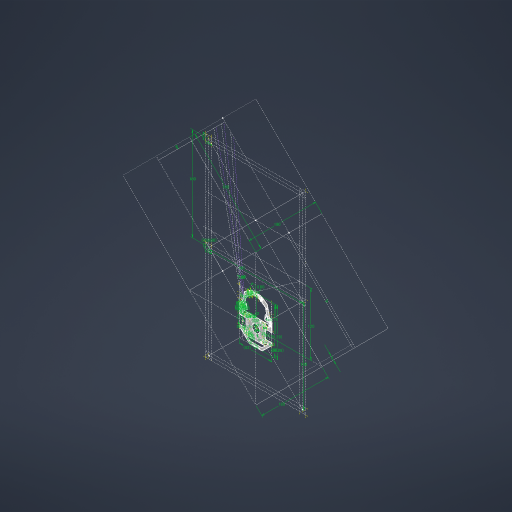
# Autodesk Inventor part: chassis
Saved by Autodesk Inventor 2023.5 (Build 275446000, 446)
## iProperties
Created: 2024-12-08
Part Number: chassis
Material: 一般
Document SubType Name: Modeling
Designer: IshiiLabHonda
Density: 1 g/cm^3
Appearance: 既定
Author: IshiiLabHonda
Autodesk Inventor part; units mm, degrees
(part 1 of 2)
ref_plane "YZ Plane" through (0, 0, 0) normal (1, 0, 0) x (0, 1, 0)
ref_plane "XZ Plane" through (0, 0, 0) normal (0, 1, 0) x (-1, 0, 0)
ref_plane "XY Plane" through (0, 0, 0) normal (0, 0, 1) x (1, 0, 0)
sketch "スケッチ1" plane through (0, 0, 0) normal (0, 0, 1) x (1, 0, 0)
  line L0 (0, 0) -> (0, 1) construction
  line L1 (0, 0) -> (1, 0) construction
  line L2 (-90, 90) -> (90, 90) construction
  line L3 (90, 90) -> (90, -90) construction
  line L4 (90, -90) -> (-90, -90) construction
  line L5 (-90, -90) -> (-90, 90) construction
  line L6 (-90, -90) -> (90, 90) construction
  line L7 (-90, 90) -> (90, -90) construction
  line L8 (-84, 96) -> (-84, 84) construction
  line L9 (-84, 84) -> (-96, 84) construction
  line L10 (-96, 84) -> (-96, 96) construction
  line L11 (-96, 96) -> (-84, 84) construction
  line L12 (-84, 96) -> (-96, 84) construction
  line L13 (-96, 96) -> (-84, 96) construction
  line L14 (-96, -96) -> (-96, -84) construction
  line L15 (-84, -96) -> (-96, -96) construction
  line L16 (-96, -96) -> (-84, -84) construction
  line L17 (-96, -84) -> (-84, -96) construction
  line L18 (-84, -84) -> (-84, -96) construction
  line L19 (-96, -84) -> (-84, -84) construction
  line L20 (96, -96) -> (84, -96) construction
  line L21 (96, -84) -> (96, -96) construction
  line L22 (96, -96) -> (84, -84) construction
  line L23 (84, -96) -> (96, -84) construction
  line L24 (84, -84) -> (96, -84) construction
  line L25 (84, -96) -> (84, -84) construction
  line L26 (96, 96) -> (96, 84) construction
  line L27 (84, 96) -> (96, 96) construction
  line L28 (96, 96) -> (84, 84) construction
  line L29 (96, 84) -> (84, 96) construction
  line L30 (84, 84) -> (84, 96) construction
  line L31 (96, 84) -> (84, 84) construction
  line L32 (-84, 84) -> (-84, -84) construction
  line L33 (-96, 84) -> (-96, -84) construction
  line L34 (-84, -84) -> (84, -84) construction
  line L35 (-84, -96) -> (84, -96) construction
  line L36 (96, 84) -> (96, -84) construction
  line L37 (84, 84) -> (84, -84) construction
  line L38 (-84, 96) -> (84, 96) construction
  line L39 (-84, 84) -> (84, 84) construction
  line L40 (-19, 15) -> (19, 15) construction
  line L41 (19, 15) -> (19, -15) construction
  line L42 (19, -15) -> (-19, -15) construction
  line L43 (-19, -15) -> (-19, 15) construction
  line L44 (-19, 15) -> (19, -15) construction
  line L45 (19, 15) -> (-19, -15) construction
  line L46 (-30.25, 11.5) -> (-19, 11.5) construction
  line L47 (-19, -11.5) -> (-30.25, -11.5) construction
  line L48 (-30.25, -11.5) -> (-30.25, 11.5) construction
  line L49 (-30.25, 11.5) -> (-19, -11.5) construction
  line L50 (-19, 11.5) -> (-30.25, -11.5) construction
  line L51 (30.25, 11.5) -> (19, 11.5) construction
  line L52 (19, -11.5) -> (30.25, -11.5) construction
  line L53 (30.25, -11.5) -> (30.25, 11.5) construction
  line L54 (30.25, 11.5) -> (19, -11.5) construction
  line L55 (19, 11.5) -> (30.25, -11.5) construction
  line L56 (-19, -10) -> (19, -10) construction
  line L57 (-19, -12.5) -> (19, -12.5) construction
  line L58 (-19, 10) -> (19, 10) construction
  line L59 (-19, 12.5) -> (19, 12.5) construction
  line L60 (-16.5, -15) -> (-16.5, 15) construction
  line L61 (16.5, -15) -> (16.5, 15) construction
  line L62 (-12.5, -10) -> (-12.5, -15) construction
  line L63 (-16.5, -10) -> (-12.5, -15) construction
  line L64 (-16.5, -15) -> (-12.5, -10) construction
  circle A0 centre (-14.5, -12.5) radius 0.8 construction
  line L65 (12.5, -10) -> (12.5, -15) construction
  line L66 (16.5, -10) -> (12.5, -15) construction
  line L67 (16.5, -15) -> (12.5, -10) construction
  circle A1 centre (14.5, -12.5) radius 0.8 construction
  line L68 (-12.5, 10) -> (-12.5, 15) construction
  line L69 (-16.5, 10) -> (-12.5, 15) construction
  line L70 (-16.5, 15) -> (-12.5, 10) construction
  circle A2 centre (-14.5, 12.5) radius 0.8 construction
  line L71 (12.5, 10) -> (12.5, 15) construction
  line L72 (16.5, 10) -> (12.5, 15) construction
  circle A3 centre (14.5, 12.5) radius 0.8 construction
  line L73 (16.5, 15) -> (12.5, 10) construction
  line L74 (-96, 276) -> (-84, 276) construction
  line L75 (-84, 276) -> (-84, 264) construction
  line L76 (-84, 264) -> (-96, 264) construction
  line L77 (-96, 264) -> (-96, 276) construction
  line L78 (-96, 276) -> (-84, 264) construction
  line L79 (-84, 276) -> (-96, 264) construction
  line L80 (-90, 90) -> (-90, 270) construction
  line L81 (-96, 264) -> (-96, 96) construction
  line L82 (-84, 264) -> (-84, 96) construction
  line L83 (96, 276) -> (84, 276) construction
  line L84 (84, 276) -> (84, 264) construction
  line L85 (84, 264) -> (96, 264) construction
  line L86 (96, 264) -> (96, 276) construction
  line L87 (96, 276) -> (84, 264) construction
  line L88 (84, 276) -> (96, 264) construction
  line L89 (90, 90) -> (90, 270) construction
  line L90 (96, 264) -> (96, 96) construction
  line L91 (84, 264) -> (84, 96) construction
  line L92 (-84, 276) -> (84, 276) construction
  line L93 (-84, 264) -> (84, 264) construction
  line L94 (-90, 270) -> (90, 270) construction
  line L95 (-90, 270) -> (90, 90) construction
  line L96 (-90, 90) -> (90, 270) construction
  circle A4 centre (0, 0) radius 15 construction
  line L97 (-96, 120) -> (96, 120) construction
  line L98 (0, 127.2792) -> (0, -127.2792) construction
  line L99 (-127.2792, 0) -> (127.2792, 0) construction
  line L100 (127.2792, 0) -> (0, -127.2792) construction
  line L101 (0, -127.2792) -> (-127.2792, 0) construction
  line L102 (-127.2792, 0) -> (0, 127.2792) construction
  line L103 (0, 127.2792) -> (127.2792, 0) construction
  line L104 (127.2792, 254.5584) -> (254.5584, 127.2792) construction
  line L105 (254.5584, 127.2792) -> (127.2792, 0) construction
  line L106 (127.2792, 0) -> (0, 127.2792) construction
  line L107 (0, 127.2792) -> (127.2792, 254.5584) construction
  line L108 (-127.2792, 254.5584) -> (0, 127.2792) construction
  line L109 (0, 127.2792) -> (-127.2792, 0) construction
  line L110 (-127.2792, 0) -> (-254.5584, 127.2792) construction
  line L111 (-254.5584, 127.2792) -> (-127.2792, 254.5584) construction
  line L112 (0, 381.8377) -> (127.2792, 254.5584) construction
  line L113 (127.2792, 254.5584) -> (0, 127.2792) construction
  line L114 (0, 127.2792) -> (-127.2792, 254.5584) construction
  line L115 (-127.2792, 254.5584) -> (0, 381.8377) construction
  line L116 (190.9188, 63.6396) -> (63.6396, 190.9188) construction
  line L117 (-190.9188, 190.9188) -> (-63.6396, 63.6396) construction
  line L118 (59.397, -59.397) -> (186.6762, 67.8823) construction
  line L119 (59.397, 186.6762) -> (186.6762, 59.397) construction
  line L120 (63.6396, 190.9188) -> (-63.6396, 318.1981) construction
  line L121 (-186.6762, 186.6762) -> (-59.397, 313.9554) construction
  point P0 (-90, -90)
  point P1 (90, -90)
  point P2 (-24.625, 0)
  point P3 (-84, 120)
  point P4 (84, 120)
  point P5 (0, 0)
  dimension "d0" = 1
  dimension "d1" = 1
  dimension "d2" = 180
  dimension "d3" = 180
  dimension "d4" = 12
  dimension "d5" = 12
  dimension "d8" = 360
  dimension "d10" = 38
  dimension "d12" = 11.25
  dimension "d13" = 23
  dimension "d14" = 5
  dimension "d15" = 2.5
  dimension "d16" = 4
  dimension "d17" = 1.6
  dimension "d22" = 12
  dimension "d23" = 12
  dimension "d24" = 180
  dimension "d25" = 25
  dimension "d26" = 30
  dimension "d27" = 30
  dimension "d29" = 120
  dimension "d331" = 180
  dimension "d334" = 180
  dimension "d337" = 180
  dimension "d340" = 6
  dimension "d341" = 6
  dimension "d342" = 6
  constraints: 244 end point, 29 point on line, 27 symmetric about line, 19 midpoint, 18 parallel, 10 perpendicular, 5 centre point, 4 coincident, 2 collinear, 1 horizontal, 1 vertical, 91 other
  measures "d0" distance of L0.start L0.end
  measures "d1" distance of L0.start L1.end
  measures "d2" distance of L2.start L2.end
  measures "d3" distance of L2.end L3.end
  measures "d4" distance of L9.end L10.end
  measures "d5" distance of L8.end L9.end
  measures "d10" distance of L40.start L40.end
  measures "d12" distance of L46.start L46.end
  measures "d13" distance of L47.end L46.start
  measures "d14" distance between parallel lines of L56 L42
  measures "d15" distance between parallel lines of L43 L60
  measures "d16" distance between parallel lines of L60 L62
  measures "d17" diameter of A0
  measures "d22" distance of L75.end L76.end
  measures "d23" distance of L76.end L74.start
  measures "d24" distance of L2.start L80.end
  measures "d25" distance between parallel lines of L57 L59
  measures "d26" distance between parallel lines of L42 L40
  measures "d27" diameter of A4
  measures "d29" distance between parallel lines of L1 L97
  measures "d331" distance of L100.start L100.end
  measures "d334" distance of L102.end L104.start
  measures "d337" distance of L102.end L108.start
  measures "d340" distance between parallel lines of L118 L105
  measures "d341" distance between parallel lines of L116 L119
  measures "d342" distance between parallel lines of L111 L121
sketch "スケッチ4" plane through (0, 0, 0) normal (0, 0, 1) x (1, 0, 0)
  line L0 (-84, 264) -> (-96, 264) construction
  line L1 (-90, 90) -> (-90, 270) construction
  line L2 (-96, 264) -> (-96, 96) construction
  line L3 (-96, 96) -> (-84, 96) construction
  line L4 (-84, 96) -> (-84, 84) construction
  line L5 (-84, 96) -> (-96, 84) construction
  line L6 (-96, 96) -> (-84, 84) construction
  line L7 (-84, 264) -> (-84, 96) construction
  line L8 (-84, 84) -> (-96, 84) construction
  line L9 (84, -84) -> (96, -84) construction
  line L10 (84, -96) -> (96, -84) construction
  line L11 (96, -96) -> (84, -84) construction
  line L12 (96, -84) -> (96, -96) construction
  line L13 (96, -96) -> (84, -96) construction
  line L14 (0, 0) -> (0, 1) construction
  line L15 (0, 0) -> (1, 0) construction
  line L16 (16.5, 15) -> (12.5, 10) construction
  line L17 (-96, 84) -> (-96, -84) construction
  line L18 (-84, 84) -> (-84, -84) construction
  line L19 (-90, -90) -> (-90, 90) construction
  line L20 (-90, 90) -> (90, 90) construction
  line L21 (-84, -84) -> (84, -84) construction
  line L22 (-84, -96) -> (84, -96) construction
  line L23 (-90, -90) -> (90, 90) construction
  line L24 (90, -90) -> (-90, -90) construction
  line L25 (-90, 90) -> (90, -90) construction
  line L26 (84, 84) -> (84, -84) construction
  line L27 (90, 90) -> (90, -90) construction
  line L28 (96, 84) -> (96, -84) construction
  line L29 (-96, 84) -> (-96, 96) construction
  line L30 (-84, -84) -> (-84, -96) construction
  line L31 (-96, -84) -> (-84, -84) construction
  line L32 (-84, -96) -> (-96, -96) construction
  line L33 (-96, -96) -> (-84, -84) construction
  line L34 (-96, -84) -> (-84, -96) construction
  line L35 (-96, -96) -> (-96, -84) construction
  line L36 (84, -96) -> (84, -84) construction
  line L37 (-19, -15) -> (-19, 15) construction
  line L38 (-30.25, 11.5) -> (-19, 11.5) construction
  line L39 (-19, -11.5) -> (-30.25, -11.5) construction
  line L40 (-19, 11.5) -> (-30.25, -11.5) construction
  line L41 (-30.25, 11.5) -> (-19, -11.5) construction
  line L42 (-30.25, -11.5) -> (-30.25, 11.5) construction
  line L43 (12.5, 10) -> (12.5, 15) construction
  circle A0 centre (14.5, 12.5) radius 0.8 construction
  line L44 (30.25, 11.5) -> (19, 11.5) construction
  line L45 (16.5, 10) -> (12.5, 15) construction
  circle A1 centre (14.5, -12.5) radius 0.8 construction
  line L46 (16.5, -15) -> (12.5, -10) construction
  line L47 (16.5, -10) -> (12.5, -15) construction
  line L48 (12.5, -10) -> (12.5, -15) construction
  circle A2 centre (-14.5, -12.5) radius 0.8 construction
  line L49 (-12.5, -10) -> (-12.5, -15) construction
  line L50 (-16.5, -15) -> (-12.5, -10) construction
  line L51 (-16.5, -10) -> (-12.5, -15) construction
  line L52 (96, 84) -> (84, 84) construction
  line L53 (96, 96) -> (96, 84) construction
  line L54 (84, 96) -> (96, 96) construction
  line L55 (96, 96) -> (84, 84) construction
  line L56 (84, 84) -> (84, 96) construction
  line L57 (96, 84) -> (84, 96) construction
  line L58 (-96, 264) -> (-96, 276) construction
  line L59 (-84, 276) -> (-84, 264) construction
  line L60 (-96, 276) -> (-84, 276) construction
  line L61 (-96, 276) -> (-84, 264) construction
  line L62 (-84, 276) -> (-96, 264) construction
  line L63 (-84, 84) -> (84, 84) construction
  line L64 (-84, 96) -> (84, 96) construction
  line L65 (84, 264) -> (84, 96) construction
  line L66 (90, 90) -> (90, 270) construction
  line L67 (-90, 90) -> (90, 270) construction
  line L68 (-90, 270) -> (90, 90) construction
  line L69 (96, 264) -> (96, 96) construction
  line L70 (-96, 120) -> (96, 120) construction
  line L71 (-84, 264) -> (84, 264) construction
  line L72 (-84, 276) -> (84, 276) construction
  line L73 (-90, 270) -> (90, 270) construction
  line L74 (84, 276) -> (84, 264) construction
  line L75 (84, 264) -> (96, 264) construction
  line L76 (96, 264) -> (96, 276) construction
  line L77 (96, 276) -> (84, 264) construction
  line L78 (96, 276) -> (84, 276) construction
  line L79 (84, 276) -> (96, 264) construction
  line L80 (-19, 15) -> (19, 15) construction
  line L81 (19, 15) -> (19, -15) construction
  line L82 (19, -15) -> (-19, -15) construction
  circle A3 centre (-14.5, 12.5) radius 0.8 construction
  line L83 (-16.5, 10) -> (-12.5, 15) construction
  line L84 (-12.5, 10) -> (-12.5, 15) construction
  line L85 (-16.5, 15) -> (-12.5, 10) construction
  circle A4 centre (0, 0) radius 15 construction
  line L86 (-19, 10) -> (19, 10) construction
  line L87 (-19, 12.5) -> (19, 12.5) construction
  line L88 (-19, 15) -> (19, -15) construction
  line L89 (19, 15) -> (-19, -15) construction
  line L90 (-19, -10) -> (19, -10) construction
  line L91 (-19, -12.5) -> (19, -12.5) construction
  line L92 (16.5, -15) -> (16.5, 15) construction
  line L93 (19, 11.5) -> (30.25, -11.5) construction
  line L94 (19, -11.5) -> (30.25, -11.5) construction
  line L95 (30.25, -11.5) -> (30.25, 11.5) construction
  line L96 (30.25, 11.5) -> (19, -11.5) construction
  line L97 (-16.5, -15) -> (-16.5, 15) construction
  line L98 (-84, 120) -> (30.25, 40.0013) construction
  line L99 (84, 120) -> (-30.25, 40.0013) construction
  line L100 (-30.25, 57) -> (30.25, 57) construction
  line L101 (1.0005, 57) -> (-30.25, 35.1182) construction
  line L102 (-1.0005, 57) -> (30.25, 35.1182) construction
  line L103 (-12.9471, 57) -> (-30.25, 44.8844) construction
  line L104 (-10.2335, 58.2897) -> (-6.2185, 52.5556) construction
  line L105 (-6.2185, 52.5556) -> (-11.543, 48.8274) construction
  line L106 (-11.543, 48.8274) -> (-15.558, 54.5615) construction
  line L107 (-15.558, 54.5615) -> (-10.2335, 58.2897) construction
  line L108 (-10.2335, 58.2897) -> (-11.543, 48.8274) construction
  line L109 (-6.2185, 52.5556) -> (-15.558, 54.5615) construction
  line L110 (-9.6599, 57.4705) -> (-14.9844, 53.7423) construction
  line L111 (-6.7921, 53.3748) -> (-12.1165, 49.6465) construction
  line L112 (-10.8882, 53.5585) -> (-10.2329, 54.0174) construction
  line L113 (-10.8882, 53.5585) -> (-10.4294, 52.9032) construction
  line L114 (-10.5199, 55.6476) -> (-8.7991, 53.1902) construction
  line L115 (-8.7991, 53.1902) -> (-11.2566, 51.4694) construction
  line L116 (-11.2566, 51.4694) -> (-12.9773, 53.9269) construction
  line L117 (-12.9773, 53.9269) -> (-10.5199, 55.6476) construction
  line L118 (-10.5199, 55.6476) -> (-11.2566, 51.4694) construction
  line L119 (-8.7991, 53.1902) -> (-12.9773, 53.9269) construction
  circle A5 centre (-10.8882, 53.5585) radius 0.8 construction
  line L120 (-30.25, 11.5) -> (-30.25, 57) construction
  line L121 (30.25, 11.5) -> (30.25, 57) construction
  line L122 (-6.1403, 52) -> (6.1403, 52) construction
  line L123 (-31, 57) -> (-31, -31) construction
  line L124 (31, 57) -> (31, -31) construction
  line L125 (-30.25, 57) -> (-31, 57) construction
  line L126 (30.25, 57) -> (31, 57) construction
  line L127 (-31, 8.5) -> (31, 8.5) construction
  line L128 (-31, -8.5) -> (31, -8.5) construction
  circle A6 centre (0, 0) radius 7.5 construction
  line L129 (-31, -31) -> (31, -31) construction
  line L130 (-30.25, 44.8844) -> (-31, 44.3592) construction
  line L131 (-30.25, 35.1182) -> (-31, 34.593) construction
  line L132 (-26.25, 26.5) -> (-26.3613, 27.2922) construction
  line L133 (-26.25, 26.5) -> (-25.4578, 26.6113) construction
  line L134 (-29.0736, 28.6277) -> (-24.1223, 29.3236) construction
  line L135 (-24.1223, 29.3236) -> (-23.4264, 24.3723) construction
  line L136 (-23.4264, 24.3723) -> (-28.3777, 23.6764) construction
  line L137 (-28.3777, 23.6764) -> (-29.0736, 28.6277) construction
  line L138 (-29.0736, 28.6277) -> (-23.4264, 24.3723) construction
  line L139 (-24.1223, 29.3236) -> (-28.3777, 23.6764) construction
  circle A7 centre (-26.25, 26.5) radius 0.8 construction
  line L140 (-26.25, 57) -> (-26.25, -31) construction
  line L141 (-96, 180) -> (96, 180) construction
  line L142 (-26.3613, 27.2922) -> (-65.7556, 307.5968) construction
  line L143 (-186.6762, 186.6762) -> (-59.397, 313.9554) construction
  line L144 (59.397, 186.6762) -> (186.6762, 59.397) construction
  line L145 (-26.25, 26.5) -> (-80.4501, 292.9022) construction
  line L146 (-26.25, 26.5) -> (-47.9742, 302.5327) construction
  line L147 (63.6396, 190.9188) -> (-63.6396, 318.1981) construction
  line L148 (10.2335, 58.2897) -> (6.2185, 52.5556) construction
  line L149 (6.2185, 52.5556) -> (11.543, 48.8274) construction
  line L150 (11.543, 48.8274) -> (15.558, 54.5615) construction
  line L151 (15.558, 54.5615) -> (10.2335, 58.2897) construction
  line L152 (10.2335, 58.2897) -> (11.543, 48.8274) construction
  line L153 (6.2185, 52.5556) -> (15.558, 54.5615) construction
  line L154 (9.6599, 57.4705) -> (14.9844, 53.7423) construction
  line L155 (6.7921, 53.3748) -> (12.1165, 49.6465) construction
  line L156 (10.8882, 53.5585) -> (10.2329, 54.0174) construction
  line L157 (10.8882, 53.5585) -> (10.4294, 52.9032) construction
  line L158 (10.5199, 55.6476) -> (8.7991, 53.1902) construction
  line L159 (8.7991, 53.1902) -> (11.2566, 51.4694) construction
  line L160 (11.2566, 51.4694) -> (12.9773, 53.9269) construction
  line L161 (12.9773, 53.9269) -> (10.5199, 55.6476) construction
  line L162 (10.5199, 55.6476) -> (11.2566, 51.4694) construction
  line L163 (8.7991, 53.1902) -> (12.9773, 53.9269) construction
  circle A8 centre (10.8882, 53.5585) radius 0.8 construction
  line L164 (-24.1223, 29.3236) -> (-19.1709, 30.0195) construction
  line L165 (-19.1709, 30.0195) -> (-18.4751, 25.0681) construction
  line L166 (-18.4751, 25.0681) -> (-23.4264, 24.3723) construction
  line L167 (-24.1223, 29.3236) -> (-29.0736, 28.6277) construction
  line L168 (-29.0736, 28.6277) -> (-28.3777, 23.6764) construction
  line L169 (-28.3777, 23.6764) -> (-23.4264, 24.3723) construction
  line L170 (28.3777, 23.6764) -> (29.0736, 28.6277) construction
  line L171 (24.1223, 29.3236) -> (19.1709, 30.0195) construction
  line L172 (19.1709, 30.0195) -> (18.4751, 25.0681) construction
  line L173 (18.4751, 25.0681) -> (23.4264, 24.3723) construction
  line L174 (24.1223, 29.3236) -> (29.0736, 28.6277) construction
  line L175 (29.0736, 28.6277) -> (28.3777, 23.6764) construction
  line L176 (28.3777, 23.6764) -> (23.4264, 24.3723) construction
  line L177 (24.1223, 29.3236) -> (28.3777, 23.6764) construction
  line L178 (23.4264, 24.3723) -> (29.0736, 28.6277) construction
  line L179 (-21.2987, 27.1959) -> (-61.3286, 312.0238) construction
  line L180 (-21.2987, 27.1959) -> (-76.2182, 297.1342) construction
  line L181 (-21.2987, 27.1959) -> (-42.5405, 297.0989) construction
  line L182 (-24.1223, 29.3236) -> (-18.4751, 25.0681) construction
  line L183 (-23.4264, 24.3723) -> (-19.1709, 30.0195) construction
  line L184 (-15.558, 54.5615) -> (-18.0155, 52.8407) construction
  line L185 (-18.0155, 52.8407) -> (-14.0004, 47.1067) construction
  line L186 (-14.0004, 47.1067) -> (-11.543, 48.8274) construction
  point P0 (90, -90)
  point P1 (-90, -90)
  point P2 (-24.625, 0)
  point P3 (0, 61.1826)
  point P4 (-5.9733, 57)
  point P5 (-8.226, 55.4227)
  point P6 (0, 180)
  point P7 (8.226, 55.4227)
  dimension "d264" = 110
  dimension "d275" = 7
  dimension "d276" = 6.5
  dimension "d277" = 5
  dimension "d278" = 3
  dimension "d279" = 3
  dimension "d280" = 1.6
  dimension "d281" = 8
  dimension "d284" = 5
  dimension "d288" = 17
  dimension "d289" = 15
  dimension "d290" = 0.75
  dimension "d291" = 0.75
  dimension "d292" = 88
  dimension "d296" = 5
  dimension "d297" = 5
  dimension "d298" = 1.6
  dimension "d299" = 8
  dimension "d345" = 7
  dimension "d346" = 15
  dimension "d356" = 16
  dimension "d367" = 4
  dimension "d369" = 42
  dimension "d370" = 6
  dimension "d371" = 62
  dimension "d382" = 5
  dimension "d385" = 7
  dimension "d513" = 3
  constraints: 172 end point, 38 point on line, 25 symmetric about line, 19 parallel, 15 perpendicular, 13 midpoint, 6 point on circle, 5 collinear, 4 centre point, 4 coincident, 2 equal length, 8 other
  measures "d264" angle of L99 L98
  measures "d275" distance of L104.start L104.end
  measures "d276" distance of L106.end L104.start
  measures "d277" distance between parallel lines of L110 L111
  measures "d278" distance of L115.end L116.end
  measures "d279" distance of L114.end L115.end
  measures "d280" diameter of A5
  measures "d281" distance between parallel lines of L101 L103
  measures "d284" distance between parallel lines of L100 L122
  measures "d288" distance between parallel lines of L128 L127
  measures "d289" diameter of A6
  measures "d290" distance between parallel lines of L123 L120
  measures "d291" distance between parallel lines of L121 L124
  measures "d292" distance between parallel lines of L129 L100
  measures "d296" distance of L135.end L136.end
  measures "d297" distance of L134.end L135.end
  measures "d298" diameter of A7
  measures "d299" angle of L140 L132
  measures "d345" angle of L145 L146
  measures "d346" distance from line of L38 L132.start
  measures "d356" distance between parallel lines of L129 L82
  measures "d367" distance between parallel lines of L120 L140
  measures "d369" distance between parallel lines of L80 L100
  measures "d370" distance of L112.start point (-5.973, 57)
  measures "d371" distance of L123.end L124.end
  measures "d382" distance of L134.end L164.end
  measures "d385" angle of L180 L181
  measures "d513" distance between parallel lines of L185 L106
sketch "スケッチ5" plane through (0, 0, 0) normal (0, 0, 1) x (1, 0, 0)
  line L0 (0, 0) -> (0, 1) construction
  line L1 (30.25, 11.5) -> (19, 11.5) construction
  line L2 (19, 11.5) -> (30.25, -11.5) construction
  line L3 (30.25, 11.5) -> (19, -11.5) construction
  line L4 (30.25, -11.5) -> (30.25, 11.5) construction
  line L5 (19, -11.5) -> (30.25, -11.5) construction
  line L6 (-90, 90) -> (90, 90) construction
  line L7 (-90, -90) -> (90, 90) construction
  line L8 (-90, 90) -> (90, -90) construction
  line L9 (-84, 84) -> (-84, -84) construction
  line L10 (-96, 84) -> (-96, -84) construction
  line L11 (-90, -90) -> (-90, 90) construction
  line L12 (-84, 84) -> (-96, 84) construction
  line L13 (-96, 84) -> (-96, 96) construction
  line L14 (84, 84) -> (84, -84) construction
  line L15 (90, 90) -> (90, -90) construction
  line L16 (96, 84) -> (84, 84) construction
  line L17 (96, 84) -> (96, -84) construction
  line L18 (90, -90) -> (-90, -90) construction
  line L19 (-84, -84) -> (84, -84) construction
  line L20 (-84, -96) -> (84, -96) construction
  line L21 (-84, -84) -> (-84, -96) construction
  line L22 (-96, -96) -> (-96, -84) construction
  line L23 (-84, -96) -> (-96, -96) construction
  line L24 (-96, -96) -> (-84, -84) construction
  line L25 (-96, -84) -> (-84, -96) construction
  line L26 (-96, -84) -> (-84, -84) construction
  line L27 (0, 0) -> (1, 0) construction
  line L28 (-84, 264) -> (-96, 264) construction
  line L29 (-96, 276) -> (-84, 276) construction
  line L30 (-96, 264) -> (-96, 276) construction
  line L31 (-84, 276) -> (-96, 264) construction
  line L32 (-96, 276) -> (-84, 264) construction
  line L33 (-84, 276) -> (-84, 264) construction
  line L34 (84, -96) -> (84, -84) construction
  line L35 (96, -96) -> (84, -96) construction
  line L36 (96, -84) -> (96, -96) construction
  line L37 (96, -96) -> (84, -84) construction
  line L38 (84, -96) -> (96, -84) construction
  line L39 (84, -84) -> (96, -84) construction
  line L40 (-19, 15) -> (19, 15) construction
  line L41 (19, 15) -> (19, -15) construction
  line L42 (16.5, 15) -> (12.5, 10) construction
  line L43 (12.5, 10) -> (12.5, 15) construction
  line L44 (16.5, 10) -> (12.5, 15) construction
  line L45 (16.5, -15) -> (16.5, 15) construction
  line L46 (-19, 10) -> (19, 10) construction
  line L47 (-19, 12.5) -> (19, 12.5) construction
  circle A0 centre (0, 0) radius 15 construction
  line L48 (-19, -10) -> (19, -10) construction
  line L49 (-19, -12.5) -> (19, -12.5) construction
  line L50 (19, -15) -> (-19, -15) construction
  line L51 (-19, 15) -> (19, -15) construction
  line L52 (19, 15) -> (-19, -15) construction
  line L53 (-16.5, -15) -> (-16.5, 15) construction
  line L54 (-19, -15) -> (-19, 15) construction
  line L55 (-30.25, 11.5) -> (-19, 11.5) construction
  line L56 (-19, -11.5) -> (-30.25, -11.5) construction
  line L57 (-30.25, -11.5) -> (-30.25, 11.5) construction
  line L58 (-30.25, 11.5) -> (-19, -11.5) construction
  line L59 (-19, 11.5) -> (-30.25, -11.5) construction
  line L60 (-12.5, 10) -> (-12.5, 15) construction
  circle A1 centre (-14.5, 12.5) radius 0.8 construction
  line L61 (-16.5, 10) -> (-12.5, 15) construction
  line L62 (-16.5, 15) -> (-12.5, 10) construction
  circle A2 centre (14.5, 12.5) radius 0.8 construction
  line L63 (-84, 96) -> (-96, 84) construction
  line L64 (-96, 96) -> (-84, 96) construction
  line L65 (-84, 96) -> (-84, 84) construction
  line L66 (-96, 96) -> (-84, 84) construction
  line L67 (-96, 264) -> (-96, 96) construction
  line L68 (-84, 264) -> (-84, 96) construction
  line L69 (-84, 96) -> (84, 96) construction
  line L70 (-84, 84) -> (84, 84) construction
  line L71 (84, 84) -> (84, 96) construction
  line L72 (96, 96) -> (96, 84) construction
  line L73 (96, 96) -> (84, 84) construction
  line L74 (96, 84) -> (84, 96) construction
  line L75 (-96, 120) -> (96, 120) construction
  line L76 (84, 96) -> (96, 96) construction
  line L77 (-84, 264) -> (84, 264) construction
  line L78 (84, 264) -> (84, 96) construction
  line L79 (-84, 276) -> (84, 276) construction
  line L80 (96, 264) -> (96, 96) construction
  line L81 (-90, 270) -> (90, 270) construction
  line L82 (-90, 270) -> (90, 90) construction
  line L83 (-90, 90) -> (90, 270) construction
  line L84 (90, 90) -> (90, 270) construction
  line L85 (-90, 90) -> (-90, 270) construction
  line L86 (84, 264) -> (96, 264) construction
  line L87 (96, 276) -> (84, 276) construction
  line L88 (96, 276) -> (84, 264) construction
  line L89 (84, 276) -> (96, 264) construction
  line L90 (96, 264) -> (96, 276) construction
  line L91 (84, 276) -> (84, 264) construction
  circle A3 centre (-14.5, -12.5) radius 0.8 construction
  line L92 (-12.5, -10) -> (-12.5, -15) construction
  line L93 (-16.5, -15) -> (-12.5, -10) construction
  line L94 (12.5, -10) -> (12.5, -15) construction
  circle A4 centre (14.5, -12.5) radius 0.8 construction
  line L95 (16.5, -15) -> (12.5, -10) construction
  line L96 (16.5, -10) -> (12.5, -15) construction
  line L97 (-16.5, -10) -> (-12.5, -15) construction
  line L98 (-12.9773, 53.9269) -> (-10.5199, 55.6476) construction
  line L99 (-8.7991, 53.1902) -> (-12.9773, 53.9269) construction
  circle A5 centre (-10.8882, 53.5585) radius 0.8 construction
  line L100 (-8.7991, 53.1902) -> (-11.2566, 51.4694) construction
  line L101 (-10.5199, 55.6476) -> (-11.2566, 51.4694) construction
  line L102 (-11.2566, 51.4694) -> (-12.9773, 53.9269) construction
  line L103 (-30.25, 44.8844) -> (-31, 44.3592) construction
  line L104 (-12.9471, 57) -> (-30.25, 44.8844) construction
  line L105 (-30.25, 57) -> (-31, 57) construction
  line L106 (-10.5199, 55.6476) -> (-8.7991, 53.1902) construction
  line L107 (-30.25, 57) -> (30.25, 57) construction
  line L108 (-6.2185, 52.5556) -> (-11.543, 48.8274) construction
  line L109 (-11.543, 48.8274) -> (-15.558, 54.5615) construction
  line L110 (-10.2335, 58.2897) -> (-6.2185, 52.5556) construction
  line L111 (1.0005, 57) -> (-30.25, 35.1182) construction
  line L112 (-1.0005, 57) -> (30.25, 35.1182) construction
  line L113 (-19, 15) -> (19, 15) construction
  line L114 (12.5, 10) -> (12.5, 15) construction
  line L115 (-19, 10) -> (19, 10) construction
  circle A6 centre (-14.5, 12.5) radius 0.8 construction
  line L116 (-12.5, 10) -> (-12.5, 15) construction
  line L117 (-16.5, 10) -> (-12.5, 15) construction
  line L118 (-16.5, 15) -> (-12.5, 10) construction
  line L119 (-19, 12.5) -> (19, 12.5) construction
  line L120 (30.25, 57) -> (31, 57) construction
  line L121 (30.25, 11.5) -> (30.25, 57) construction
  line L122 (-6.1403, 52) -> (6.1403, 52) construction
  line L123 (-30.25, 35.1182) -> (-31, 34.593) construction
  line L124 (-30.25, 11.5) -> (-30.25, 57) construction
  line L125 (-6.7921, 53.3748) -> (-12.1165, 49.6465) construction
  line L126 (-10.8882, 53.5585) -> (-10.4294, 52.9032) construction
  line L127 (-10.8882, 53.5585) -> (-10.2329, 54.0174) construction
  line L128 (-6.2185, 52.5556) -> (-15.558, 54.5615) construction
  line L129 (-9.6599, 57.4705) -> (-14.9844, 53.7423) construction
  line L130 (-15.558, 54.5615) -> (-10.2335, 58.2897) construction
  line L131 (-10.2335, 58.2897) -> (-11.543, 48.8274) construction
  line L132 (-30.25, 11.5) -> (-19, 11.5) construction
  line L133 (-30.25, 11.5) -> (-19, -11.5) construction
  line L134 (30.25, 11.5) -> (19, 11.5) construction
  line L135 (30.25, -11.5) -> (30.25, 11.5) construction
  line L136 (19, 11.5) -> (30.25, -11.5) construction
  line L137 (30.25, 11.5) -> (19, -11.5) construction
  line L138 (0, 0) -> (0, 1) construction
  line L139 (0, 0) -> (1, 0) construction
  circle A7 centre (0, 0) radius 7.5 construction
  circle A8 centre (0, 0) radius 15 construction
  line L140 (-16.5, -15) -> (-16.5, 15) construction
  circle A9 centre (14.5, 12.5) radius 0.8 construction
  line L141 (-12.5, -10) -> (-12.5, -15) construction
  line L142 (12.5, -10) -> (12.5, -15) construction
  line L143 (16.5, 10) -> (12.5, 15) construction
  line L144 (-16.5, -15) -> (-12.5, -10) construction
  line L145 (16.5, -10) -> (12.5, -15) construction
  line L146 (16.5, 15) -> (12.5, 10) construction
  line L147 (-19, -12.5) -> (19, -12.5) construction
  line L148 (19, -15) -> (-19, -15) construction
  line L149 (-19, 11.5) -> (-30.25, -11.5) construction
  line L150 (19, -11.5) -> (30.25, -11.5) construction
  line L151 (-19, -11.5) -> (-30.25, -11.5) construction
  line L152 (-30.25, -11.5) -> (-30.25, 11.5) construction
  line L153 (16.5, -15) -> (16.5, 15) construction
  line L154 (19, 15) -> (19, -15) construction
  line L155 (-19, -15) -> (-19, 15) construction
  line L156 (-19, 15) -> (19, -15) construction
  line L157 (19, 15) -> (-19, -15) construction
  line L158 (-31, -8.5) -> (31, -8.5) construction
  line L159 (-31, 8.5) -> (31, 8.5) construction
  line L160 (-31, -31) -> (31, -31) construction
  line L161 (-31, 57) -> (-31, -31) construction
  line L162 (31, 57) -> (31, -31) construction
  line L163 (84, -84) -> (96, -84) construction
  line L164 (84, -96) -> (96, -84) construction
  line L165 (96, -96) -> (84, -84) construction
  line L166 (96, -84) -> (96, -96) construction
  line L167 (96, -96) -> (84, -96) construction
  line L168 (-96, 84) -> (-96, -84) construction
  line L169 (-84, 84) -> (-84, -84) construction
  line L170 (-90, -90) -> (-90, 90) construction
  line L171 (-84, -84) -> (84, -84) construction
  line L172 (-84, -96) -> (84, -96) construction
  line L173 (-90, -90) -> (90, 90) construction
  line L174 (90, -90) -> (-90, -90) construction
  line L175 (-90, 90) -> (90, -90) construction
  line L176 (84, 84) -> (84, -84) construction
  line L177 (90, 90) -> (90, -90) construction
  line L178 (96, 84) -> (96, -84) construction
  line L179 (84, -96) -> (84, -84) construction
  line L180 (-19, -10) -> (19, -10) construction
  circle A10 centre (14.5, -12.5) radius 0.8 construction
  line L181 (16.5, -15) -> (12.5, -10) construction
  line L182 (-16.5, -10) -> (-12.5, -15) construction
  line L183 (-84, -84) -> (-84, -96) construction
  line L184 (-96, -84) -> (-84, -84) construction
  line L185 (-84, -96) -> (-96, -96) construction
  line L186 (-96, -96) -> (-84, -84) construction
  line L187 (-96, -84) -> (-84, -96) construction
  line L188 (-96, -96) -> (-96, -84) construction
  circle A11 centre (-14.5, -12.5) radius 0.8 construction
  line L189 (-96, 96) -> (-84, 96) construction
  line L190 (-84, 96) -> (-84, 84) construction
  line L191 (-84, 96) -> (-96, 84) construction
  line L192 (-96, 96) -> (-84, 84) construction
  line L193 (84, 96) -> (96, 96) construction
  line L194 (96, 84) -> (84, 84) construction
  line L195 (96, 96) -> (96, 84) construction
  line L196 (96, 96) -> (84, 84) construction
  line L197 (96, 84) -> (84, 96) construction
  line L198 (-96, 120) -> (96, 120) construction
  line L199 (-84, 96) -> (84, 96) construction
  line L200 (-90, 90) -> (90, 90) construction
  line L201 (-84, 84) -> (-96, 84) construction
  line L202 (-96, 84) -> (-96, 96) construction
  line L203 (-84, 84) -> (84, 84) construction
  line L204 (84, 120) -> (-30.25, 40.0013) construction
  line L205 (-84, 120) -> (30.25, 40.0013) construction
  line L206 (84, 84) -> (84, 96) construction
  line L207 (-84, 264) -> (-96, 264) construction
  line L208 (-90, 90) -> (-90, 270) construction
  line L209 (-96, 264) -> (-96, 96) construction
  line L210 (-84, 264) -> (-84, 96) construction
  line L211 (96, 264) -> (96, 96) construction
  line L212 (84, 264) -> (84, 96) construction
  line L213 (90, 90) -> (90, 270) construction
  line L214 (-90, 90) -> (90, 270) construction
  line L215 (-90, 270) -> (90, 90) construction
  line L216 (-84, 264) -> (84, 264) construction
  line L217 (-90, 270) -> (90, 270) construction
  line L218 (-96, 264) -> (-96, 276) construction
  line L219 (-96, 276) -> (-84, 276) construction
  line L220 (-96, 276) -> (-84, 264) construction
  line L221 (-84, 276) -> (-96, 264) construction
  line L222 (-84, 276) -> (-84, 264) construction
  line L223 (-84, 276) -> (84, 276) construction
  line L224 (84, 264) -> (96, 264) construction
  line L225 (96, 264) -> (96, 276) construction
  line L226 (96, 276) -> (84, 264) construction
  line L227 (96, 276) -> (84, 276) construction
  line L228 (84, 276) -> (96, 264) construction
  line L229 (84, 276) -> (84, 264) construction
  line L230 (-31, 8.5) -> (-19, 8.5)
  line L231 (-31, -8.5) -> (-19, -8.5)
  line L232 (-19, 8.5) -> (-19, -8.5)
  circle A12 centre (0, 0) radius 7.5
  line L233 (31, 8.5) -> (19, 8.5)
  line L234 (31, -8.5) -> (19, -8.5)
  line L235 (19, 8.5) -> (19, -8.5)
  line L236 (31, 8.5) -> (31, 8.5)
  line L237 (-31, -8.5) -> (-12.1203, -31) construction
  line L238 (-12.1203, -31) -> (12.1203, -31)
  line L239 (31, -8.5) -> (12.1203, -31) construction
  circle A13 centre (-14.5, 12.5) radius 1.05
  circle A14 centre (14.5, 12.5) radius 1.05
  circle A15 centre (-14.5, -12.5) radius 1.05
  circle A16 centre (14.5, -12.5) radius 1.05
  line L240 (-26.25, 26.5) -> (-26.3613, 27.2922) construction
  line L241 (-26.25, 26.5) -> (-25.4578, 26.6113) construction
  circle A17 centre (-26.25, 26.5) radius 0.8 construction
  line L242 (-24.1223, 29.3236) -> (-23.4264, 24.3723) construction
  line L243 (-28.3777, 23.6764) -> (-29.0736, 28.6277) construction
  line L244 (-24.1223, 29.3236) -> (-28.3777, 23.6764) construction
  line L245 (-29.0736, 28.6277) -> (-24.1223, 29.3236) construction
  line L246 (-23.4264, 24.3723) -> (-28.3777, 23.6764) construction
  line L247 (-29.0736, 28.6277) -> (-23.4264, 24.3723) construction
  line L248 (-29.0736, 28.6277) -> (-28.3777, 23.6764)
  line L249 (-24.1223, 29.3236) -> (-19.1709, 30.0195) construction
  line L250 (-19.1709, 30.0195) -> (-18.4751, 25.0681) construction
  line L251 (-18.4751, 25.0681) -> (-23.4264, 24.3723) construction
  line L252 (28.3777, 23.6764) -> (23.4264, 24.3723) construction
  line L253 (18.4751, 25.0681) -> (23.4264, 24.3723) construction
  line L254 (19.1709, 30.0195) -> (18.4751, 25.0681) construction
  line L255 (24.1223, 29.3236) -> (19.1709, 30.0195) construction
  line L256 (24.1223, 29.3236) -> (29.0736, 28.6277) construction
  line L257 (29.0736, 28.6277) -> (28.3777, 23.6764) construction
  line L258 (-29.0736, 28.6277) -> (-19.1709, 30.0195)
  line L259 (-18.4751, 25.0681) -> (-19.1709, 30.0195)
  line L260 (-18.4751, 25.0681) -> (-28.3777, 23.6764)
  line L261 (19.1709, 30.0195) -> (29.0736, 28.6277)
  line L262 (28.3777, 23.6764) -> (29.0736, 28.6277)
  line L263 (28.3777, 23.6764) -> (18.4751, 25.0681)
  line L264 (19.1709, 30.0195) -> (18.4751, 25.0681)
  line L265 (-9.6771, 59.2897) -> (9.6771, 59.2897)
  line L266 (-9.6771, 59.2897) -> (-9.6771, 59.2897)
  line L267 (-3.6771, 59.2897) -> (-0.9296, 58.2897)
  line L268 (-0.9296, 58.2897) -> (0.9296, 58.2897)
  line L269 (0.9296, 58.2897) -> (3.6771, 59.2897)
  line L270 (-4.6137, 54.2897) -> (4.6137, 54.2897)
  line L271 (-18.1736, 44.795) -> (-4.6137, 54.2897)
  line L272 (-31, 8.5) -> (-22.0451, 50.6295)
  line L273 (-22.0451, 50.6295) -> (-9.6771, 59.2897)
  line L274 (31, 8.5) -> (22.0451, 50.6295)
  line L275 (-18.1736, 44.795) -> (-23.6565, 19)
  line L276 (18.1736, 44.795) -> (23.6565, 19)
  line L277 (-23.6565, 19) -> (23.6565, 19)
  line L278 (-17.6308, -20) -> (17.6308, -20)
  line L279 (17.6308, -20) -> (11.5077, -26)
  line L280 (11.5077, -26) -> (-11.5077, -26)
  line L281 (-11.5077, -26) -> (-17.6308, -20)
  line L282 (-31, -8.5) -> (-31, -12.5)
  line L283 (-31, -12.5) -> (-12.1203, -31)
  line L284 (31, -8.5) -> (31, -12.5)
  line L285 (31, -12.5) -> (12.1203, -31)
  line L286 (-31, 8.5) -> (-31, 26.5)
  line L287 (-31, 26.5) -> (-26.3435, 30.4073)
  line L288 (31, 8.5) -> (31, 26.5)
  line L289 (31, 26.5) -> (26.3435, 30.4073)
  line L290 (-8.1203, -31) -> (-6.6203, -29.5)
  line L291 (-6.6203, -29.5) -> (6.6203, -29.5)
  line L292 (6.6203, -29.5) -> (8.1203, -31)
  line L293 (18.1736, 44.795) -> (4.6137, 54.2897)
  line L294 (22.0451, 50.6295) -> (9.6771, 59.2897)
  line L295 (-23.6565, 19) -> (-24.8255, 13.5)
  line L296 (-24.8255, 13.5) -> (-20.8255, 13.5)
  line L297 (-20.8255, 13.5) -> (-15.3255, 19)
  line L298 (23.6565, 19) -> (24.8255, 13.5)
  line L299 (24.8255, 13.5) -> (20.8255, 13.5)
  line L300 (20.8255, 13.5) -> (15.3255, 19)
  line L301 (-17.6308, -20) -> (-24.2643, -13.5)
  line L302 (-24.2643, -13.5) -> (-21.2643, -13.5)
  line L303 (-21.2643, -13.5) -> (-11.6308, -20)
  line L304 (17.6308, -20) -> (24.2643, -13.5)
  line L305 (24.2643, -13.5) -> (21.2643, -13.5)
  line L306 (21.2643, -13.5) -> (11.6308, -20)
  circle A18 centre (-10.1308, -17) radius 0.625 construction
  circle A19 centre (-10.1308, -17) radius 0.8
  circle A20 centre (-10.1308, -17) radius 1.5
  line L307 (-11.6308, -20) -> (-11.6308, -15) construction
  circle A21 centre (10.1308, -17) radius 0.625 construction
  circle A22 centre (10.1308, -17) radius 0.8
  circle A23 centre (10.1308, -17) radius 1.5
  circle A24 centre (-9, 15.5) radius 0.625 construction
  circle A25 centre (-9, 15.5) radius 0.8
  circle A26 centre (-9, 15.5) radius 1.5
  circle A27 centre (9, 15.5) radius 0.625 construction
  circle A28 centre (9, 15.5) radius 0.8
  circle A29 centre (9, 15.5) radius 1.5
  circle A30 centre (-21.0348, 43.3585) radius 0.8
  circle A31 centre (-21.0348, 43.3585) radius 1.5 construction
  circle A32 centre (21.0348, 43.3585) radius 0.475 construction
  circle A33 centre (21.0348, 43.3585) radius 0.8
  circle A34 centre (21.0348, 43.3585) radius 1.5 construction
  line L308 (-30.8721, 30.6471) -> (-17.9987, 32.4563)
  line L309 (-17.9987, 32.4563) -> (-16.6765, 23.0488)
  line L310 (-16.6765, 23.0488) -> (-29.55, 21.2395)
  line L311 (-29.55, 21.2395) -> (-30.8721, 30.6471)
  line L312 (-22.0451, 50.6295) -> (-18.1736, 44.795) construction
  line L313 (-21.8107, 27.6837) -> (-26, 24.1685)
  line L314 (-26, 24.1685) -> (-26, 13.5)
  line L315 (-24.8255, 13.5) -> (-26, 13.5)
  line L316 (21.8107, 27.6837) -> (26, 24.1685)
  line L317 (26, 24.1685) -> (26, 13.5)
  line L318 (24.8255, 13.5) -> (26, 13.5)
  circle A35 centre (-28.5, 18.5) radius 0.475 construction
  circle A36 centre (-28.5, 18.5) radius 0.8
  circle A37 centre (-28.5, 18.5) radius 1.5
  circle A38 centre (28.5, 18.5) radius 0.8
  circle A39 centre (28.5, 18.5) radius 1.5
  circle A40 centre (28.5, 18.5) radius 0.475 construction
  line L319 (-12.9471, 57) -> (12.9471, 57)
  line L320 (30.8721, 30.6471) -> (17.9987, 32.4563)
  line L321 (17.9987, 32.4563) -> (16.6765, 23.0488)
  line L322 (16.6765, 23.0488) -> (29.55, 21.2395)
  line L323 (29.55, 21.2395) -> (30.8721, 30.6471)
  line L324 (-23.4801, 43.8782) -> (-18.5894, 42.8387) construction
  line L325 (-20.1093, 47.7123) -> (-28.4441, 8.5) construction
  line L326 (-13.2559, 53.976) -> (-10.4708, 55.9262)
  line L327 (-10.4708, 55.9262) -> (-8.5206, 53.1411)
  line L328 (-8.5206, 53.1411) -> (-11.3057, 51.1909)
  line L329 (-11.3057, 51.1909) -> (-13.2559, 53.976)
  line L330 (-13.2559, 53.976) -> (-8.5206, 53.1411) construction
  line L331 (-10.4708, 55.9262) -> (-11.3057, 51.1909) construction
  line L332 (13.2559, 53.976) -> (10.4708, 55.9262)
  line L333 (10.4708, 55.9262) -> (8.5206, 53.1411)
  line L334 (8.5206, 53.1411) -> (11.3057, 51.1909)
  line L335 (11.3057, 51.1909) -> (13.2559, 53.976)
  circle A41 centre (-10.8882, 53.5585) radius 1.05
  circle A42 centre (10.8882, 53.5585) radius 1.05
  point P0 (-90, -90)
  point P1 (90, -90)
  point P2 (-24.625, 0)
  point P3 (-8.226, 55.4227)
  point P4 (-5.9733, 57)
  point P5 (0, 61.1826)
  point P6 (-24.625, 0)
  point P7 (-90, -90)
  point P8 (90, -90)
  point P9 (-5.9733, 57)
  point P10 (5.9733, 57)
  point P11 (12.9773, 53.9269)
  point P12 (8.7991, 53.1902)
  point P13 (26.3435, 30.4073)
  point P14 (11.6308, -20)
  point P15 (0, 57.9513)
  point P16 (21.8107, 27.6837)
  dimension "d352" = 15
  dimension "d359" = 2.1
  dimension "d360" = 2.1
  dimension "d361" = 2.1
  dimension "d362" = 2.1
  dimension "d405" = 1
  dimension "d410" = 1
  dimension "d411" = 6
  dimension "d412" = 20
  dimension "d413" = 5
  dimension "d414" = 1.5
  dimension "d422" = 12
  dimension "d426" = 5
  dimension "d427" = 4
  dimension "d428" = 5
  dimension "d430" = 5
  dimension "d432" = 50
  dimension "d434" = 4
  dimension "d435" = 4
  dimension "d436" = 130
  dimension "d437" = 18
  dimension "d438" = 4
  dimension "d439" = 1.5
  dimension "d451" = 4
  dimension "d466" = 5
  dimension "d467" = 45
  dimension "d468" = 4
  dimension "d469" = 5
  dimension "d470" = 3
  dimension "d471" = 6
  dimension "d491" = 1.25
  dimension "d492" = 1.6
  dimension "d497" = 3
  dimension "d499" = 3
  dimension "d503" = 1.25
  dimension "d504" = 1.6
  dimension "d505" = 3
  dimension "d506" = 3.5
  dimension "d507" = 9
  dimension "d509" = 1.6
  dimension "d510" = 3
  dimension "d515" = 1.5
  dimension "d516" = 1.5
  dimension "d517" = 2.25
  dimension "d518" = 2.25
  dimension "d520" = 5
  dimension "d521" = 5
  dimension "d532" = 0.95
  dimension "d533" = 1.6
  dimension "d534" = 3
  dimension "d538" = 2.5
  dimension "d539" = 5
  dimension "d546" = 90.2897
  dimension "d547" = 9.5
  dimension "d548" = 13
  dimension "d549" = 59.2897
  dimension "d552" = 2
  dimension "d556" = 0.2
  dimension "d557" = 0.2
  dimension "d562" = 2.1
  constraints: 178 end point, 49 horizontal alignment, 30 centre point, 23 point on line, 21 coincident, 20 parallel, 12 equal radius, 9 perpendicular, 8 collinear, 4 midpoint, 2 horizontal, 1 equal length, 1 tangent, 1 vertical, 43 other
  measures "d352" diameter of A12
  measures "d359" diameter of A13
  measures "d360" diameter of A14
  measures "d361" diameter of A15
  measures "d362" diameter of A16
  measures "d405" distance from line of L265 L110.start
  measures "d410" distance between parallel lines of L268 L265
  measures "d411" distance of L266.end L267.start
  measures "d412" angle of L267 L265
  measures "d413" distance between parallel lines of L270 L265
  measures "d414" distance between parallel lines of L271 L100
  measures "d422" angle of L161 L272
  measures "d426" distance between parallel lines of L272 L275
  measures "d428" distance between parallel lines of L280 L238
  measures "d432" angle of L158 L237
  measures "d434" distance of L158.start L282.end
  measures "d435" distance of L158.end L284.end
  measures "d436" angle of L286 L287
  measures "d437" distance of L159.start L286.end
  measures "d438" distance of L237.end L290.start
  measures "d439" distance between parallel lines of L160 L291
  measures "d451" distance between parallel lines of L283 L281
  measures "d466" distance between parallel lines of L159 L296
  measures "d467" angle of L297 L277
  measures "d468" distance of L295.end L296.end
  measures "d469" distance between parallel lines of L302 L231
  measures "d470" distance of L301.end L302.end
  measures "d471" distance of L278.start L303.end
  measures "d491" diameter of A18
  measures "d492" diameter of A19
  measures "d497" diameter of A20
  measures "d499" distance from line of L278 A18.centre
  measures "d503" diameter of A24
  measures "d504" diameter of A25
  measures "d505" diameter of A26
  measures "d506" distance from line of L277 A24.centre
  measures "d509" diameter of A30
  measures "d510" diameter of A31
  measures "d515" distance between parallel lines of L250 L309
  measures "d516" distance between parallel lines of L311 L243
  measures "d517" distance between parallel lines of L246 L310
  measures "d518" distance between parallel lines of L308 L258
  measures "d520" distance between parallel lines of L313 L287
  measures "d521" distance between parallel lines of L161 L314
  measures "d532" diameter of A35
  measures "d533" diameter of A36
  measures "d534" diameter of A37
  measures "d538" distance from line of L161 A35.centre
  measures "d539" distance from line of L315 A35.centre
  measures "d546" distance between parallel lines of L238 L265
  measures "d547" distance between parallel lines of L310 L308
  measures "d548" distance between parallel lines of L309 L311
  measures "d549" distance of the line from the sketch origin of L265
  measures "d552" distance from line of L324 L271.start
  measures "d556" distance between parallel lines of L98 L326
  measures "d557" distance between parallel lines of L329 L102
  measures "d562" diameter of A41
extrude "押し出し10" add sketch "スケッチ5" against normal blind 1 contours L272 A37 L310 L314 L315 L296 L297 L277 L300 L299 L318 L317 L322 L274 A39 L233 L235 L234 L284 L285 L238 L292 L291 L290 L283 L282 L231 L232 L230 | L272 A36 A37 | L272 A36 | L272 L260 L314 L310 | L272 L258 L275 L313 L314 L260 | L314 L260 L275 L310 | L310 L275 L295 L315 L314 | L308 L275 L258 L272 | L272 L273 L319 L294 L274 L320 L276 L293 L270 L271 L275 L308 | L314 L313 L275 L260 | L290 L291 L292 L238 | L277 L297 L296 L295 | L273 L265 L267 L268 L269 L294 L319 | L277 L298 L299 L300 | L265 L269 L268 L267 | L276 L322 L317 L318 L298 | L274 L261 L276 L320 | L276 L263 L317 L322 | L276 L316 L317 L263 | L317 L263 L274 L322 | L274 L263 L317 L316 L276 L261 | L274 A38 A39 | L274 A38 | L301 L302 L303 L278 | L306 L305 L304 L278 | A19 | A20 | A22 | A23 | A25 | A26 | A28 | A29 | A30 | A33 | L326 L327 L328 L329 | L335 L334 L333 L332 | A41 | A42 picked at (-27.2535, 18.6745) picked at (-28.5231, 18.309) picked at (27.2634, 18.2699) picked at (28.2668, 18.7302)
extrude "押し出し11" cut sketch "スケッチ5" against normal blind 1.5 contours L277 L297 L296 L295 | L277 L298 L299 L300 | L301 L302 L303 L278 | L306 L305 L304 L278
chamfer "面取り8" distance 2 angle 45 2 edges at (-24.8255, 13.5, -0.5) (24.8255, 13.5, -0.5)
chamfer "面取り9" distance 1 angle 45 2 edges at (-24.2643, -13.5, -0.5) (24.2643, -13.5, -0.5)
extrude "押し出し12" add sketch "スケッチ5" against normal blind 1 contours L286 L287 L311 L310 L272 A37 | A37 L272 A36 | A36 L272 | L287 L248 L260 L272 L310 L311 | L287 L258 L272 L260 L248 | L287 L272 L258 | L289 L261 L274 | L261 L289 L262 L263 L274 | L323 L322 L274 L263 L262 L289 | L289 L288 L274 A39 L322 L323 | A39 L274 A38 | A38 L274 picked at (-29.7367, 18.7298) picked at (-29.0023, 18.5094) picked at (29.203, 17.4555) picked at (29.0402, 18.5343)
chamfer "面取り10" distance 2 angle 45 2 edges at (-31, 8.5, -0.5) (31, 8.5, -0.5)
chamfer "面取り11" distance 0.8 angle 45 2 edges at (-31, -8.5, -0.5) (31, -8.5, -0.5)
extrude "押し出し13" cut sketch "スケッチ5" against normal blind 1.5 contours A19 | A22 | A25 | A28
extrude "押し出し14" cut sketch "スケッチ5" against normal blind 1.5 contours A30 | A33
extrude "押し出し15" cut sketch "スケッチ5" against normal blind 1.5 contours L314 L260 L275 L310 | L310 L275 L295 L315 L314 | L314 L313 L275 L260 | L277 L297 L296 L295
chamfer "面取り12" distance 2 angle 45 1 edges at (-26, 13.5, -0.5)
extrude "押し出し16" cut sketch "スケッチ5" against normal blind 1.5 contours L277 L298 L299 L300 | L276 L322 L317 L318 L298 | L276 L263 L317 L322 | L276 L316 L317 L263
chamfer "面取り13" distance 2 angle 45 1 edges at (26, 13.5, -0.5)